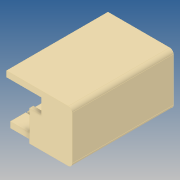
# Autodesk Inventor part: Case_Body
Saved by Autodesk Inventor 2020 (Build 240168000, 168)
## iProperties
Created: 2019-02-19
Part Number: Case_Body
Material: 일반
Document SubType Name: Modeling
Designer: Jeong Ji Hoon
Density: 1 g/cm^3
Appearance: 베이지색
Author: Jeong Ji Hoon
## iProperties of the stored document _3D 인쇄.ipt
Created: 2019-08-13
Part Number: _3D 인쇄
Material: 일반
Document SubType Name: Modeling
Designer: Jeong Ji Hoon
Density: 1 g/cm^3
Appearance: 기본값
Author: Jeong Ji Hoon
Autodesk Inventor part; units mm, degrees
ref_plane "YZ Plane" through (0, 0, 0) normal (1, 0, 0) x (0, 1, 0)
ref_plane "XZ Plane" through (0, 0, 0) normal (0, 1, 0) x (-1, 0, 0)
ref_plane "XY Plane" through (0, 0, 0) normal (0, 0, 1) x (1, 0, 0)
sketch "스케치1" plane through (0, 0, 0) normal (0, 0, 1) x (1, 0, 0)
  line L0 (0, 0) -> (18.6, 0)
  line L1 (18.6, 0) -> (18.6, 13.5)
  line L2 (18.6, 13.5) -> (0, 13.5)
  line L3 (0, 13.5) -> (0, 0)
  line L4 (1.5, 12) -> (17.1, 12)
  line L5 (17.1, 12) -> (17.1, 1.5)
  line L6 (17.1, 1.5) -> (1.5, 1.5)
  line L7 (1.5, 1.5) -> (1.5, 12)
  dimension "d4" = 18.6
  dimension "d5" = 13.5
  dimension "d6" = 1.5
  constraints: 16 end point, 4 parallel, 2 perpendicular, 1 horizontal, 3 other
  measures "d4" distance of L2.end L1.end
  measures "d5" distance of L0.end L1.end
  measures "d6" distance between parallel lines of L2 L4
extrude "돌출1" add sketch "스케치1" along normal blind 25.5
sketch "스케치2" plane through (0, 0, 25.5) normal (0, 0, 1) x (1, 0, 0)
  line L0 (0, 0) -> (18.6, 0) projected
  line L1 (18.6, 0) -> (18.6, 13.5) projected
  line L2 (0, 0) -> (18.6, 0)
  line L3 (18.6, 0) -> (18.6, 8)
  line L4 (18.6, 8) -> (0, 8)
  line L5 (18.6, 13.5) -> (0, 13.5) projected
  line L6 (18.6, 8) -> (10.6, 8)
  line L7 (10.6, 8) -> (10.6, 13.5)
  line L8 (10.6, 13.5) -> (18.6, 13.5)
  line L9 (18.6, 13.5) -> (18.6, 8)
  line L10 (0, 13.5) -> (0, 0) projected
  line L11 (17.1, 12) -> (1.5, 12) projected
  line L12 (0, 13.5) -> (10.6, 13.5)
  line L13 (10.6, 13.5) -> (10.6, 12)
  line L14 (10.6, 12) -> (0, 12)
  line L15 (0, 12) -> (0, 13.5)
  line L16 (1.5, 1.5) -> (1.5, 12) projected
  line L17 (7.5, 8) -> (7.5, 0)
  point P0 (0, 12)
  dimension "d9" = 8
  dimension "d14" = 8
  dimension "d58" = 6
  constraints: 24 end point, 6 point on line, 5 parallel, 4 perpendicular, 3 horizontal
  measures "d9" distance between parallel lines of L0 L4
  measures "d14" distance between parallel lines of L1 L7
  measures "d58" distance between parallel lines of L16 L17
extrude "돌출2" add sketch "스케치2" along normal blind 1 contours L17 L4 L1 L0 | L10 L5 L7 L11 L14 | L4 L7 L5 L1
sketch "스케치3" plane through (0, 0, 0) normal (0, 0, -1) x (-1, 0, 0)
  line L0 (-17.1, 1.5) -> (-17.1, 12) projected
  line L1 (-17.1, 12) -> (-1.5, 12) projected
  line L2 (-1.5, 12) -> (-1.5, 1.5) projected
  line L3 (-1.5, 1.5) -> (-17.1, 1.5) projected
  line L4 (0, 0) -> (-18.6, 0) projected
  line L5 (0, 13.5) -> (0, 0) projected
  line L6 (-18.6, 13.5) -> (0, 13.5) projected
  line L7 (-18.6, 0) -> (-18.6, 13.5) projected
  line L8 (-18.6, 13.5) -> (0, 13.5) projected
  line L9 (0, 0) -> (-1.5, 0)
  line L10 (-1.5, 0) -> (-1.5, 13.5)
  line L11 (-1.5, 13.5) -> (0, 13.5)
  line L12 (0, 13.5) -> (0, 0)
  point P0 (-1.5, 6.75)
  constraints: 8 end point, 2 parallel, 1 horizontal, 1 midpoint, 1 perpendicular, 1 point on line, 1 vertical alignment
extrude "돌출3" cut sketch "스케치3" against normal up to next contours L2 L10 L6 L5 L4
sketch "스케치4" plane through (18.6, 0, 0) normal (0, -1, 0) x (1, 0, 0)
  line L0 (-7.8, 21) -> (-17.1, 21)
  line L1 (-17.1, 21) -> (-17.1, 21.5)
  line L2 (-17.1, 21.5) -> (-7.8, 21.5)
  line L3 (-7.8, 21.5) -> (-7.8, 21)
  line L4 (-17.1, 25.5) -> (-17.1, 0) projected
  line L5 (-11.1, 26.5) -> (0, 26.5) projected
  point P0 (-18.6, 0)
  point P1 (-17.1, 26.5)
  dimension "d17" = 0.5
  dimension "d18" = 9.3
  dimension "d19" = 5
  constraints: 8 end point, 2 parallel, 1 collinear, 1 horizontal, 1 perpendicular
  measures "d17" distance of L0.end L1.end
  measures "d18" distance of L0.start L0.end
  measures "d19" distance between parallel lines of L2 L5
extrude "돌출4" cut sketch "스케치4" against normal up to next
fillet "모깎기1" radius 1 2 edges at (18.6, 13.5, 13.25) (18.6, 0, 13.25)
sketch "스케치11" plane through (1.5, 12, 0) normal (-1, 0, 0) x (0, 0, 1)
  line L0 (1, 0.75) -> (2, 0.75)
  line L1 (2, 0.75) -> (2, -11.25)
  line L2 (2, -11.25) -> (1, -11.25)
  line L3 (1, -11.25) -> (1, 0.75)
  line L4 (0, -10.5) -> (0, 0) projected
  line L5 (0, 1.5) -> (26.5, 1.5) projected
  line L6 (21, -12) -> (0, -12) projected
  dimension "d43" = 1
  dimension "d44" = 1
  dimension "d45" = 0.75
  dimension "d46" = 0.75
  constraints: 8 end point, 2 parallel, 1 horizontal, 1 perpendicular
  measures "d43" distance of L1.end L2.end
  measures "d44" distance between parallel lines of L4 L3
  measures "d45" distance between parallel lines of L5 L0
  measures "d46" distance between parallel lines of L2 L6
extrude "돌출8" cut sketch "스케치11" against normal blind 16.1
equation "\"d6\" = t"
equation "\"t\" = 1.5"
